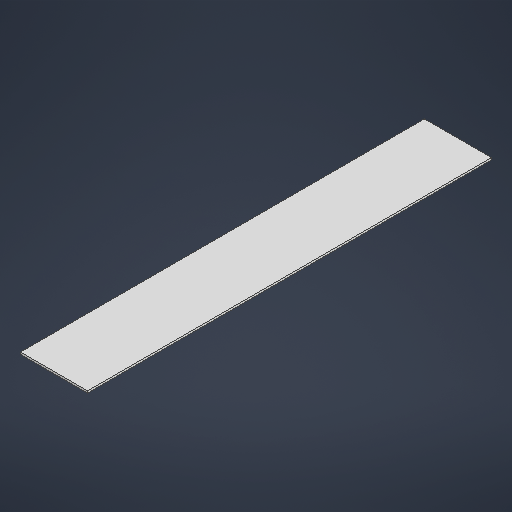
# Autodesk Inventor part: recta
Saved by Autodesk Inventor 2027 (Build 310192060, 192F)
## iProperties
Created: 2026-09-04
Part Number: recta
Material: Genérico
Document SubType Name: Modeling
Designer: Leandro
Density: 1 g/cm^3
Appearance: Valor por defecto
Author: Leandro
Autodesk Inventor part; units mm, degrees
ref_plane "YZ Plane" through (0, 0, 0) normal (1, 0, 0) x (0, 1, 0)
ref_plane "XZ Plane" through (0, 0, 0) normal (0, 1, 0) x (-1, 0, 0)
ref_plane "XY Plane" through (0, 0, 0) normal (0, 0, 1) x (1, 0, 0)
sketch "Boceto1" plane through (0, 0, 0) normal (0, 1, 0) x (-1, 0, 0)
  line L0 (1.7078, -28.1982) -> (51.7078, -28.1982)
  line L1 (51.7078, -28.1982) -> (51.7078, 272.8018)
  line L2 (1.7078, -28.1982) -> (1.7078, 272.8018)
  line L3 (1.7078, 272.8018) -> (51.7078, 272.8018)
  point P0 (0, 0)
  dimension "d2" = 50
  dimension "d3" = 301
  dimension "d4" = 301
  constraints: 8 end point, 1 horizontal, 1 perpendicular, 1 vertical
  measures "d2" distance of L0.start L0.end
  measures "d3" distance of L0.end L1.end
  measures "d4" distance of L0.start L2.end
extrude "Extrusión1" add sketch "Boceto1" along normal mid plane 1.5
